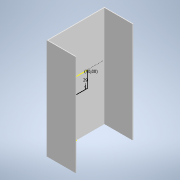
# Autodesk Inventor part: Caja
Saved by Autodesk Inventor 2021 (Build 250183000, 183)
## iProperties
Created: 2022-11-24
Part Number: Caja
Material: Genérico
Document SubType Name: Modeling
Designer: sergi
Density: 1 g/cm^3
Appearance: Valor por defecto
Author: sergi
Autodesk Inventor part; units mm, degrees
ref_plane "YZ Plane" through (0, 0, 0) normal (1, 0, 0) x (0, 1, 0)
ref_plane "XZ Plane" through (0, 0, 0) normal (0, 1, 0) x (-1, 0, 0)
ref_plane "XY Plane" through (0, 0, 0) normal (0, 0, 1) x (1, 0, 0)
sketch "Boceto1" plane through (0, 0, 0) normal (0, 1, 0) x (-1, 0, 0)
  line L0 (-53, -53) -> (53, -53)
  line L1 (53, -53) -> (53, 53)
  line L2 (53, 53) -> (-53, 53)
  line L3 (-53, 53) -> (-53, -53)
  line L4 (-53, -53) -> (53, 53) construction
  line L5 (53, -53) -> (-53, 53) construction
  point P0 (0, 0)
  dimension "d0" = 106
  dimension "d1" = 106
  constraints: 12 end point, 2 midpoint, 2 parallel, 1 horizontal, 1 perpendicular
  measures "d0" distance of L2.end L1.end
  measures "d1" distance of L1.end L0.end
extrude "Extrusión1" add sketch "Boceto1" along normal blind 185
shell "Vaciado1" thickness 1.5 removed faces 2 at (17.6667, 0, -17.6667) at (17.6667, 185, -17.6667)
split "Dividir1" plane through (0, 0, 0) removes the side toward (1, 0, 0)
sketch "Boceto2" plane through (-51.5, 0, -51.5) normal (1, 0, 0) x (0, 0, -1)
  line L0 (-71.9943, 102) -> (-31.0057, 102) projected
  line L1 (-31.0057, 102) -> (-31.0057, 73)
  line L2 (-31.0057, 102) -> (-2.0057, 102) construction
  line L3 (-31.0057, 73) -> (-71.9943, 73)
  line L4 (-71.9943, 73) -> (-71.9943, 102)
  line L5 (-31.0057, 102) -> (-32.0057, 102)
  line L6 (-32.0057, 102) -> (-71.0057, 102)
  line L7 (-71.0057, 102) -> (-71.0057, 73)
  line L8 (-71.0057, 73) -> (-32.0057, 73)
  line L9 (-32.0057, 73) -> (-32.0057, 102)
  point P0 (-51.5, 0)
  dimension "d5" = 29
  dimension "d6" = 90
  dimension "d8" = 1
  dimension "d9" = 39
  dimension "d10" = 29
  constraints: 18 end point, 4 perpendicular, 2 horizontal, 2 parallel, 1 point on line, 1 vertical
  measures "d5" distance of L0.end L1.end
  measures "d6" angle of L1 L2
  measures "d8" distance of L0.end L5.end
  measures "d9" distance of L8.end L7.end
  measures "d10" distance of L7.end L6.end
extrude "Extrusión2" cut sketch "Boceto2" against normal blind 10 contours L0 L9 L3 L7
